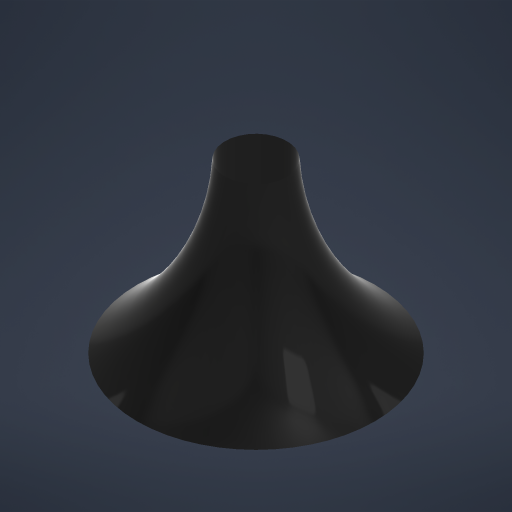
# Autodesk Inventor part: aufhaengung_ende
Saved by Autodesk Inventor 2023 (Build 270158000, 158)
## iProperties
Created: 2022-06-26
Part Number: aufhaengung_ende
Material: Generic
Document SubType Name: Modeling
Designer: bananenbrot
Density: 1 g/cm^3
Appearance: Default
Author: bananenbrot
Autodesk Inventor part; units mm, degrees
ref_plane "YZ Plane" through (0, 0, 0) normal (1, 0, 0) x (0, 1, 0)
ref_plane "XZ Plane" through (0, 0, 0) normal (0, 1, 0) x (-1, 0, 0)
ref_plane "XY Plane" through (0, 0, 0) normal (0, 0, 1) x (1, 0, 0)
sketch "Sketch1" plane through (0, 0, 0) normal (1, 0, 0) x (0, 1, 0)
  spline S0 degree 2 poles (144.5465, -57.8242) (146.4589, -59.529) (148.3712, -61.2338) knots 0.397376 0.397376 0.397376 0.909763 0.909763 0.909763 weights 0.999998 0.999997 0.999998
  spline S1 degree 3 poles (148.3712, -61.2338) (145.4357, -63.9958) (142.1284, -66.5479) (133.9847, -71.7297) (129.2192, -73.8866) (122.6716, -75.6215) (120.5117, -75.911) (117.5795, -75.8038) (116.4784, -75.6403) (114.7831, -75.0056) (114.1405, -74.649) (113.0617, -73.7127) (112.6451, -73.1713) (112.1633, -72.1987) (112.0293, -71.8331) (111.9289, -71.4578) knots -3.269118 -3.269118 -3.269118 -3.269118 -2.559935 -2.559935 -1.5672 -1.5672 -1.008898 -1.008898 -0.686053 -0.686053 -0.465554 -0.465554 -0.257093 -0.257093 -0.139706 -0.139706 -0.139706 -0.139706
  spline S2 degree 3 poles (111.9289, -71.4578) (112.6966, -70.9881) (113.4597, -70.5117) (123.0587, -64.396) (131.3801, -57.7603) (138.4898, -50.0803) knots -8.986295 -8.986295 -8.986295 -8.986295 -8.71793 -8.71793 -5.588526 -5.588526 -5.588526 -5.588526
  spline S3 degree 2 poles (138.4898, -50.0803) (142.1005, -53.2991) (145.711, -56.5179) knots 0.224389 0.224389 0.224389 1.191797 1.191797 1.191797 weights 0.999996 0.999988 0.999996
  line L0 (145.711, -56.5179) -> (144.5465, -57.8242)
  spline S4 degree 2 poles (153.8176, -55.372) (151.8438, -53.6123) (149.87, -51.8527) knots 0.391675 0.391675 0.391675 0.920526 0.920526 0.920526 weights 0.999998 0.999997 0.999998
  line L1 (149.87, -51.8527) -> (148.7055, -53.159)
  spline S5 degree 2 poles (148.7055, -53.159) (145.089, -49.9348) (141.4723, -46.7105) knots 0.223527 0.223527 0.223527 1.192553 1.192553 1.192553 weights 0.999996 0.999988 0.999996
  spline S6 degree 3 poles (141.4723, -46.7105) (147.1872, -39.9492) (151.9575, -32.4291) (158.3139, -16.5141) (159.9807, -8.4349) (159.9998, -0.1442) knots -5.139674 -5.139674 -5.139674 -5.139674 -2.489358 -2.489358 -0.002056 -0.002056 -0.002056 -0.002056
  spline S7 degree 3 poles (159.9998, -0.1442) (159.9998, -0.1389) (159.9999, -0.1336) (160, -0.0858) (160, -0.0434) (160, -0.0006) (160, -0.0003) (160, 0) knots -0.014334 -0.014334 -0.014334 -0.014334 -0.012741 -0.012741 0 0 0.00009 0.00009 0.00009 0.00009
  spline S8 degree 3 poles (160, 0) (160, 0.0003) (160, 0.0006) (160, 0.0434) (160, 0.0858) (159.9999, 0.1364) (159.9998, 0.1446) (159.9998, 0.1527) knots -0.025663 -0.025663 -0.025663 -0.025663 -0.025573 -0.025573 -0.012832 -0.012832 -0.010394 -0.010394 -0.010394 -0.010394
  spline S9 degree 3 poles (159.9998, 0.1527) (159.9873, 5.2601) (159.349, 10.3143) (156.8538, 20.4053) (154.9768, 25.3486) (151.104, 33.0257) (149.4237, 35.8779) (147.5826, 38.6258) knots -14.294543 -14.294543 -14.294543 -14.294543 -12.453936 -12.453936 -10.549031 -10.549031 -9.356599 -9.356599 -9.356599 -9.356599
  spline S10 degree 3 poles (147.5826, 38.6258) (147.379, 38.9295) (147.1735, 39.232) (146.9661, 39.5332) knots -1.789353 -1.789353 -1.789353 -1.789353 -1.679608 -1.679608 -1.679608 -1.679608
  spline S11 degree 3 poles (146.9661, 39.5332) (146.998, 39.5385) (147.0299, 39.5437) (147.139, 39.5614) (147.2162, 39.5737) (147.4152, 39.6047) (147.5369, 39.6232) (148.019, 39.6939) (148.3758, 39.7413) (149.3903, 39.8648) (150.0305, 39.9297) (150.6862, 39.9928) knots -0.377268 -0.377268 -0.377268 -0.377268 -0.367554 -0.367554 -0.344046 -0.344046 -0.307003 -0.307003 -0.197614 -0.197614 0 0 0 0
  arc A0 (187.9088, 29.7865) -> (150.6862, 39.9928) centre (155.884, -14.0298) ccw
  arc A1 (187.9088, 29.7865) -> (220.9222, 38.7731) centre (200.8273, 47.4616) ccw
  line L2 (220.9222, 38.7731) -> (220.9222, 10.6)
  line L3 (220.9222, 10.6) -> (220.4222, 10.1)
  line L4 (220.4222, 10.1) -> (180.9222, 10.1)
  line L5 (180.9222, 10.1) -> (180.9222, 7.85)
  line L6 (180.9222, 7.85) -> (220.4222, 7.85)
  line L7 (220.4222, 7.85) -> (220.9222, 7.35)
  line L8 (220.9222, 7.35) -> (220.9222, -7.35)
  line L9 (220.9222, -7.35) -> (220.4222, -7.85)
  line L10 (220.4222, -7.85) -> (180.9222, -7.85)
  line L11 (180.9222, -7.85) -> (180.9222, -10.1)
  line L12 (180.9222, -10.1) -> (220.4222, -10.1)
  line L13 (220.4222, -10.1) -> (220.9222, -10.6)
  line L14 (220.9222, -10.6) -> (220.9222, -38.7731)
  arc A2 (220.9222, -38.7731) -> (187.9088, -29.7865) centre (200.8273, -47.4616) ccw
  arc A3 (169.9254, -38.3944) -> (187.9088, -29.7865) centre (155.884, 14.0298) ccw
  spline S12 degree 3 poles (169.9254, -38.3944) (167.9887, -38.9131) (166.1731, -39.8112) (163.0398, -42.2306) (161.7393, -43.7133) (160.7596, -45.4036) knots -1.187529 -1.187529 -1.187529 -1.187529 -0.586112 -0.586112 0 0 0 0
  spline S13 degree 3 poles (160.7596, -45.4036) (160.6302, -45.6268) (160.4996, -45.8494) (158.1975, -49.7271) (155.8837, -52.872) (153.8176, -55.372) knots -4.034725 -4.034725 -4.034725 -4.034725 -4.012891 -4.012891 -3.653746 -3.653746 -3.653746 -3.653746
  line L15 (232.9325, 0) -> (277.0212, 0)
  line L16 (220.9222, 10.1) -> (220.9222, 38.7731)
  line L17 (220.9222, 10.1) -> (275.8629, 10.1)
  arc A4 (220.9222, 38.7731) -> (275.8629, 10.1) centre (279.8258, 84.6659) ccw
  point P0 (0, 0)
  point P1 (220.9222, 10.6)
  constraints: 36 end point, 10 point on circle, 6 horizontal, 5 centre point, 5 vertical, 1 collinear, 1 vertical alignment, 87 other
revolve "Revolution1" add sketch "Sketch1" angle 360 about axis through (0, 232.9325, 0) along (0, 1, 0) contours A4 L17 L16 L2
chamfer "Chamfer1" distance 0.5 angle 45 1 edges at (0, 220.9222, -10.1)
body "Solid1"
